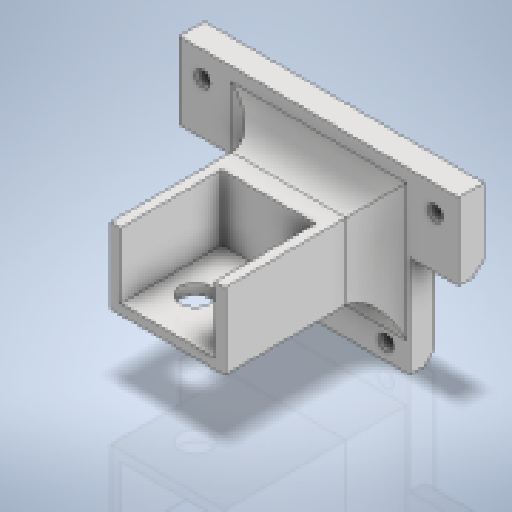
# Autodesk Inventor part: bloco_aquecimento
Saved by Autodesk Inventor 2024.3 (Build 283343000, 343)
## iProperties
Created: 2024-03-27
Part Number: bloco_aquecimento
Material: Genérico
Document SubType Name: Modeling
Designer: joaov
Density: 1 g/cm^3
Appearance: Padrão
Author: joaov
Autodesk Inventor part; units mm, degrees
ref_plane "YZ Plane" through (0, 0, 0) normal (1, 0, 0) x (0, 1, 0)
ref_plane "XZ Plane" through (0, 0, 0) normal (0, 1, 0) x (-1, 0, 0)
ref_plane "XY Plane" through (0, 0, 0) normal (0, 0, 1) x (1, 0, 0)
sketch "Esboço1" plane through (0, 0, 0) normal (0, 0, 1) x (1, 0, 0)
  line L0 (75.9001, -29.3373) -> (75.9001, -14.1373)
  line L1 (75.9001, -14.1373) -> (20.5381, -14.1373)
  line L2 (20.5381, -14.1373) -> (20.5381, -29.3373)
  line L3 (20.5381, -29.3373) -> (30.2191, -29.3373)
  line L4 (30.2191, -29.3373) -> (30.2191, -49.4373)
  line L5 (30.2191, -49.4373) -> (66.2191, -49.4373)
  line L6 (66.2191, -49.4373) -> (66.2191, -29.3373)
  line L7 (66.2191, -29.3373) -> (75.9001, -29.3373)
  line L8 (48.2191, -14.1373) -> (48.2191, -19.1373)
  line L9 (48.2191, -49.4373) -> (48.2191, -46.2373)
  line L10 (20.5381, -19.1373) -> (23.7381, -19.1373)
  line L11 (23.7381, -19.1373) -> (25.2381, -19.1373)
  line L12 (30.2191, -46.2373) -> (33.4191, -46.2373)
  line L13 (33.4191, -46.2373) -> (34.9191, -46.2373)
  circle A0 centre (25.2381, -19.1373) radius 1.5
  circle A1 centre (34.9191, -46.2373) radius 1.5
  circle A2 centre (71.2001, -19.1373) radius 1.5
  circle A3 centre (61.5191, -46.2373) radius 1.5
  point P0 (0, 0)
  dimension "d9" = 15.2
  dimension "d10" = 55.362
  dimension "d11" = 15.2
  dimension "d12" = 9.681
  dimension "d13" = 20.1
  dimension "d14" = 36
  dimension "d15" = 20.1
  dimension "d16" = 5
  dimension "d17" = 3.2
  dimension "d18" = 3.2
  dimension "d19" = 1.5
  dimension "d20" = 3.2
  dimension "d21" = 1.5
  constraints: 28 end point, 7 perpendicular, 4 point on line, 3 vertical, 2 centre point, 2 coincident, 2 horizontal alignment, 2 midpoint, 2 symmetric about line, 1 horizontal, 6 other
  measures "d9" distance of L0.start L0.end
  measures "d10" distance of L0.end L1.end
  measures "d11" distance of L1.end L2.end
  measures "d12" distance of L2.end L3.end
  measures "d13" distance of L3.end L4.end
  measures "d14" distance of L4.end L5.end
  measures "d15" distance of L5.end L6.end
  measures "d16" distance of L8.start L8.end
  measures "d17" distance of L9.start L9.end
  measures "d18" distance of L10.start L10.end
  measures "d19" distance of L10.end L11.end
  measures "d20" distance of L12.start L12.end
  measures "d21" distance of L12.end L13.end
extrude "Extrusão1" add sketch "Esboço1" along normal blind 5
sketch "Esboço2" plane through (0, 0, 5) normal (0, 0, 1) x (1, 0, 0)
  line L0 (75.9001, -14.1373) -> (20.5381, -14.1373) projected
  line L1 (30.2191, -49.4373) -> (66.2191, -49.4373) projected
  line L2 (66.2191, -49.4373) -> (66.2191, -29.3373) projected
  line L3 (38.9191, -29.3373) -> (38.9191, -22.8373)
  line L4 (57.5191, -29.3373) -> (57.5191, -35.8373)
  line L5 (57.5191, -22.8373) -> (57.5191, -35.8373)
  line L6 (57.5191, -35.8373) -> (38.9191, -35.8373)
  line L7 (38.9191, -35.8373) -> (38.9191, -22.8373)
  line L8 (38.9191, -22.8373) -> (36.9191, -22.8373)
  line L9 (36.9191, -22.8373) -> (36.9191, -35.8373)
  line L10 (36.9191, -35.8373) -> (36.9191, -37.8373)
  line L11 (36.9191, -37.8373) -> (57.5191, -37.8373)
  line L12 (57.5191, -37.8373) -> (59.5191, -37.8373)
  line L13 (59.5191, -37.8373) -> (59.5191, -22.8373)
  line L14 (59.5191, -22.8373) -> (57.5191, -22.8373)
  point P0 (0, 0)
  point P1 (30.2191, -29.3373)
  dimension "d28" = 2
  dimension "d29" = 2
  dimension "d30" = 2
  constraints: 24 end point, 4 perpendicular, 3 point on line, 2 parallel, 2 vertical
  measures "d28" distance of L3.end L8.end
  measures "d29" distance of L9.end L10.end
  measures "d30" distance of L11.end L12.end
extrude "Extrusão2" add sketch "Esboço2" along normal blind 30
sketch "Esboço3" plane through (0, 0, 5) normal (0, 0, 1) x (1, 0, 0)
  line L0 (38.9191, -35.8373) -> (38.9191, -22.8373) projected
  line L1 (38.9191, -22.8373) -> (57.5191, -22.8373)
  line L2 (57.5191, -22.8373) -> (57.5191, -35.8373)
  line L3 (57.5191, -35.8373) -> (38.9191, -35.8373)
  line L4 (38.9191, -35.8373) -> (38.9191, -22.8373)
  point P0 (0, 0)
  constraints: 8 end point, 2 parallel, 1 horizontal, 1 perpendicular
extrude "Extrusão3" add sketch "Esboço3" along normal blind 10
sketch "Esboço4" plane through (38.9191, -35.8373, 35) normal (0, 1, 0) x (1, 0, 0)
  line L0 (-2, 0) -> (20.6, 0) projected
  line L1 (9.3, 0) -> (9.3, 20)
  line L2 (18.6, 20) -> (0, 20) projected
  line L3 (0.2146, 9.9142) -> (3, 8.8)
  line L4 (3, 8.8) -> (6, 8.8)
  circle A0 centre (6, 8.8) radius 3
  line L5 (6, 10) -> (6, 8.8)
  point P0 (-38.9191, 35)
  dimension "d36" = 3
  dimension "d37" = 3
  dimension "d38" = 1.2
  constraints: 8 end point, 2 midpoint, 1 centre point, 1 coincident, 1 horizontal, 1 vertical
  measures "d36" distance of L3.start L3.end
  measures "d37" distance of L3.end L4.end
  measures "d38" distance of L5.start L5.end
extrude "Extrusão4" cut sketch "Esboço4" against normal blind 10
fillet "Arredondamento1" radius 6 4 edges at (36.9191, -30.3373, 5) (48.2191, -22.8373, 5) (59.5191, -30.3373, 5) (48.2191, -37.8373, 5)
sketch "Esboço5" plane through (20.5381, -29.3373, 0) normal (-1, 0, 0) x (0, 0, 1)
  line L0 (0, 0) -> (5, 0) projected
  line L1 (0, 0) -> (0, 2.1)
  line L2 (0, 15.2) -> (0, 0) projected
  line L3 (0, 0) -> (0, -20.1) projected
  line L4 (0, 0) -> (2.1, 0)
  line L5 (2.1, 0) -> (0, 2.1)
  point P0 (0, 29.3373)
  dimension "d42" = 2.1
  dimension "d43" = 2.1
  constraints: 6 end point, 2 point on line
  measures "d42" distance of L0.start L1.end
  measures "d43" distance of L0.start L4.end
extrude "Extrusão5" cut sketch "Esboço5" against normal blind 9.681
sketch "Esboço6" plane through (75.9001, -29.3373, 0) normal (1, 0, 0) x (0, 0, -1)
  line L0 (0, 2.1) -> (-2.1, 0) projected
  line L1 (0, 2.1) -> (0, 0)
  line L2 (0, -20.1) -> (0, 2.1) projected
  line L3 (0, 0) -> (-2.1, 0)
  line L4 (0, 2.1) -> (-2.1, 0)
  point P0 (0, 29.3373)
  dimension "d46" = 2.1
  constraints: 6 end point, 1 collinear, 1 point on line
  measures "d46" distance of L0.start L1.end
extrude "Extrusão6" cut sketch "Esboço6" against normal blind 9.681
sketch "Esboço7" plane through (66.2191, -49.4373, 5) normal (1, 0, 0) x (0, 0, -1)
  line L0 (5, 0) -> (0, 0) projected
  line L1 (5, 0) -> (5, 2.1)
  line L2 (5, 0) -> (5, 22.2) projected
  line L3 (5, 0) -> (2.9, 0)
  line L4 (2.9, 0) -> (5, 2.1)
  point P0 (5, 49.4373)
  dimension "d49" = 2.1
  dimension "d50" = 2.1
  constraints: 6 end point, 2 point on line
  measures "d49" distance of L0.start L1.end
  measures "d50" distance of L0.start L3.end
extrude "Extrusão7" cut sketch "Esboço7" against normal through all
sketch "Esboço8" plane through (20.5381, -14.1373, 0) normal (0, 1, 0) x (1, 0, 0)
  line L0 (0, -5) -> (9.681, -5) projected
  line L1 (0, -5) -> (0.1, -5)
  line L2 (0.1, -5) -> (-0.0713, -5)
  line L3 (-0.0713, -5) -> (-0.0713, 0.2754)
  line L4 (-0.0713, 0.2754) -> (0.1, 0.2754)
  line L5 (0.1, 0.2754) -> (0.1, -5)
  line L6 (55.362, -5) -> (55.262, -5)
  line L7 (55.362, -5) -> (0, -5) projected
  line L8 (55.262, -5) -> (55.4822, -5)
  line L9 (55.4822, -5) -> (55.4822, 0.1017)
  line L10 (55.4822, 0.1017) -> (55.262, 0.1017)
  line L11 (55.262, 0.1017) -> (55.262, -5)
  point P0 (-20.5381, 0)
  dimension "d53" = 0.1
  dimension "d54" = 0.1
  constraints: 20 end point, 4 parallel, 2 horizontal, 2 perpendicular, 2 point on line
  measures "d53" distance of L0.start L1.end
  measures "d54" distance of L6.start L6.end
extrude "Extrusão8" cut sketch "Esboço8" against normal blind 15.2
sketch "Esboço9" plane through (30.2191, -49.4373, 5) normal (0, -1, 0) x (1, 0, 0)
  line L0 (36, -2.9) -> (36, 0) projected
  line L1 (36, 0) -> (35.9, 0)
  line L2 (45.581, 0) -> (-9.581, 0) projected
  line L3 (35.9, 0) -> (36.1068, 0)
  line L4 (36.1068, 0) -> (36.1068, -5.0668)
  line L5 (36.1068, -5.0668) -> (35.9, -5.0668)
  line L6 (35.9, -5.0668) -> (35.9, 0)
  line L7 (3.6802, -5) -> (0, -5) projected
  line L8 (0, -5) -> (0.1, -5)
  line L9 (0.1, -5) -> (-0.0853, -5)
  line L10 (-0.0853, -5) -> (-0.0853, 0.1044)
  line L11 (-0.0853, 0.1044) -> (0.1, 0.1044)
  line L12 (0.1, 0.1044) -> (0.1, -5)
  point P0 (-30.2191, -5)
  dimension "d57" = 0.1
  dimension "d58" = 0.1
  constraints: 20 end point, 4 parallel, 2 horizontal, 2 perpendicular, 2 point on line
  measures "d57" distance of L0.end L1.end
  measures "d58" distance of L7.end L8.end
extrude "Extrusão9" cut sketch "Esboço9" against normal blind 20.1
sketch "Esboço10" plane through (66.1191, -49.4373, 5) normal (1, 0, 0) x (0, 0, -1)
  line L0 (0, 0) -> (2.9, 0) projected
  line L1 (0, 0) -> (0, 0.1)
  line L2 (0, 20.1) -> (0, 0) projected
  line L3 (0, 0.1) -> (3.2291, 0.1)
  line L4 (3.2291, 0.1) -> (3.2291, -0.3139)
  line L5 (3.2291, -0.3139) -> (0, -0.3139)
  line L6 (0, -0.3139) -> (0, 0.1)
  point P0 (5, 49.4373)
  dimension "d61" = 0.1
  constraints: 10 end point, 2 parallel, 1 horizontal, 1 perpendicular, 1 point on line
  measures "d61" distance of L0.start L1.end
extrude "Extrusão10" cut sketch "Esboço10" against normal blind 35.801
sketch "Esboço11" plane through (75.8001, -14.1373, 5) normal (1, 0, 0) x (0, 0, -1)
  line L0 (5, -15.2) -> (0, -15.2) projected
  line L1 (0, -15.2) -> (0, -15.1)
  line L2 (0, 0) -> (0, -15.2) projected
  line L3 (0, -15.1) -> (5.2297, -15.1)
  line L4 (5.2297, -15.1) -> (5.2297, -15.4949)
  line L5 (5.2297, -15.4949) -> (0, -15.4949)
  line L6 (0, -15.4949) -> (0, -15.1)
  point P0 (5, 14.1373)
  dimension "d65" = 0.1
  constraints: 10 end point, 2 parallel, 1 horizontal, 1 perpendicular, 1 point on line
  measures "d65" distance of L0.end L1.end
extrude "Extrusão11" cut sketch "Esboço11" against normal blind 9.681
sketch "Esboço12" plane through (20.6381, -14.1373, 0) normal (-1, 0, 0) x (0, 0, 1)
  line L0 (5, 0) -> (5, -15.2) projected
  line L1 (5, -15.2) -> (5, -15.1)
  line L2 (5, -15.1) -> (-0.3189, -15.1)
  line L3 (-0.3189, -15.1) -> (-0.3189, -15.5919)
  line L4 (-0.3189, -15.5919) -> (5, -15.5919)
  line L5 (5, -15.5919) -> (5, -15.1)
  point P0 (0, 14.1373)
  dimension "d68" = 0.1
  constraints: 10 end point, 2 parallel, 1 horizontal, 1 perpendicular, 1 point on line
  measures "d68" distance of L0.end L1.end
extrude "Extrusão12" cut sketch "Esboço12" against normal blind 9.681
sketch "Esboço13" plane through (20.6381, -14.1373, 0) normal (-1, 0, 0) x (0, 0, 1)
  line L0 (5, 0) -> (5, -15.1) projected
  line L1 (5, 0) -> (5, -0.1)
  line L2 (5, -0.1) -> (-1.4486, -0.1)
  line L3 (-1.4486, -0.1) -> (-1.4486, 0.7057)
  line L4 (-1.4486, 0.7057) -> (5, 0.7057)
  line L5 (5, 0.7057) -> (5, -0.1)
  point P0 (0, 14.1373)
  dimension "d71" = 0.1
  constraints: 10 end point, 2 parallel, 1 horizontal, 1 perpendicular, 1 point on line
  measures "d71" distance of L0.start L1.end
extrude "Extrusão13" cut sketch "Esboço13" against normal blind 55.162
chamfer "Chanfro1" distance 1 angle 45 4 edges at (69.7001, -19.1373, 5) (23.7381, -19.1373, 5) (33.4191, -46.2373, 5) (60.0191, -46.2373, 5)
